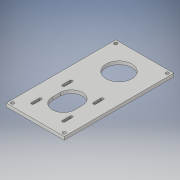
# Autodesk Inventor part: lid
Saved by Autodesk Inventor 2018 (Build 220112000, 112)
## iProperties
Created: 2018-07-04
Part Number: lid
Material: Generic
Document SubType Name: Modeling
Designer: Cole Tucker
Density: 1 g/cm^3
Appearance: Default
Author: Cole Tucker
Autodesk Inventor part; units mm, degrees
ref_plane "YZ Plane" through (0, 0, 0) normal (1, 0, 0) x (0, 1, 0)
ref_plane "XZ Plane" through (0, 0, 0) normal (0, 1, 0) x (-1, 0, 0)
ref_plane "XY Plane" through (0, 0, 0) normal (0, 0, 1) x (1, 0, 0)
sketch "Sketch1" plane through (0, 0, 0) normal (0, 1, 0) x (-1, 0, 0)
  line L0 (0, 0) -> (57.15, 0)
  line L1 (57.15, 0) -> (57.15, -107.95)
  line L2 (57.15, -107.95) -> (0, -107.95)
  line L3 (0, -107.95) -> (0, 0)
  line L4 (57.15, -53.975) -> (0, -53.975) construction
  circle A0 centre (28.575, -35.56) radius 11.049
  line L5 (28.575, -35.56) -> (43.815, -35.56) construction
  line L6 (43.815, -35.56) -> (43.815, -50.8) construction
  line L7 (43.815, -50.8) -> (28.575, -50.8) construction
  line L8 (28.575, -50.8) -> (28.575, -35.56) construction
  line L9 (28.575, -35.56) -> (13.335, -35.56) construction
  line L10 (13.335, -35.56) -> (13.335, -20.32) construction
  line L11 (13.335, -20.32) -> (28.575, -20.32) construction
  line L12 (28.575, -20.32) -> (28.575, -35.56) construction
  line L13 (43.815, -50.8) -> (13.335, -50.8) construction
  line L14 (13.335, -50.8) -> (13.335, -20.32) construction
  line L15 (13.335, -20.32) -> (43.815, -20.32) construction
  line L16 (43.815, -20.32) -> (43.815, -50.8) construction
  circle A1 centre (43.815, -50.8) radius 1.27
  circle A2 centre (43.815, -20.32) radius 1.27
  circle A3 centre (13.335, -50.8) radius 1.27
  circle A4 centre (13.335, -20.32) radius 1.27
  line L17 (28.575, -107.95) -> (28.575, -53.975) construction
  line L18 (28.575, -35.56) -> (28.575, -27.94) construction
  circle A5 centre (28.575, -27.94) radius 11.049
  line L19 (43.815, -50.8) -> (43.815, -43.18) construction
  line L20 (13.335, -50.8) -> (13.335, -43.18) construction
  line L21 (13.335, -20.32) -> (13.335, -12.7) construction
  line L22 (43.815, -20.32) -> (43.815, -12.7) construction
  circle A6 centre (43.815, -43.18) radius 1.27
  circle A7 centre (13.335, -43.18) radius 1.27
  circle A8 centre (13.335, -12.7) radius 1.27
  circle A9 centre (43.815, -12.7) radius 1.27
  line L23 (45.085, -43.18) -> (45.085, -50.8)
  line L24 (42.545, -43.18) -> (42.545, -50.8)
  line L25 (14.605, -43.18) -> (14.605, -50.8)
  line L26 (12.065, -43.18) -> (12.065, -50.8)
  line L27 (12.065, -12.7) -> (12.065, -20.32)
  line L28 (14.605, -20.32) -> (14.605, -12.7)
  line L29 (45.085, -12.7) -> (45.085, -20.32)
  line L30 (42.545, -20.32) -> (42.545, -12.7)
  line L31 (28.575, -107.95) -> (28.575, -82.55) construction
  circle A10 centre (28.575, -82.55) radius 12.7
  line L32 (57.15, 0) -> (57.15, -12.7)
  line L33 (57.15, 0) -> (44.45, 0)
  line L34 (44.45, 0) -> (57.15, -12.7) construction
  line L35 (57.15, 0) -> (50.8, -6.35) construction
  line L36 (0, 0) -> (12.7, 0) construction
  line L37 (0, 0) -> (0, -12.7) construction
  line L38 (0, -12.7) -> (12.7, 0) construction
  line L39 (0, 0) -> (6.35, -6.35) construction
  line L40 (57.15, -107.95) -> (57.15, -95.25) construction
  line L41 (57.15, -107.95) -> (44.45, -107.95) construction
  line L42 (44.45, -107.95) -> (57.15, -95.25) construction
  line L43 (57.15, -107.95) -> (50.8, -101.6) construction
  line L44 (0, -107.95) -> (12.7, -107.95) construction
  line L45 (0, -107.95) -> (0, -95.25) construction
  line L46 (0, -95.25) -> (12.7, -107.95) construction
  line L47 (6.35, -101.6) -> (0, -107.95) construction
  circle A11 centre (53.975, -104.775) radius 1.5875
  circle A12 centre (3.175, -104.775) radius 1.5875
  circle A13 centre (53.975, -3.175) radius 1.5875
  circle A14 centre (3.175, -3.175) radius 1.5875
  line L48 (17.526, -35.56) -> (17.526, -27.94)
  line L49 (39.624, -35.56) -> (39.624, -27.94)
  point P0 (38.7216, -23.5665)
  point P1 (18.4284, -23.5665)
  dimension "d0" = 57.15
  dimension "d1" = 107.95
  dimension "d2" = 22.098
  dimension "d3" = 15.24
  dimension "d4" = 15.24
  dimension "d5" = 15.24
  dimension "d6" = 15.24
  dimension "d7" = 2.54
  dimension "d8" = 2.54
  dimension "d9" = 2.54
  dimension "d10" = 2.54
  dimension "d11" = 7.62
  dimension "d12" = 22.098
  dimension "d13" = 7.62
  dimension "d14" = 7.62
  dimension "d15" = 7.62
  dimension "d16" = 7.62
  dimension "d17" = 2.54
  dimension "d18" = 2.54
  dimension "d19" = 2.54
  dimension "d20" = 2.54
  dimension "d21" = 25.4
  dimension "d22" = 25.4
  dimension "d25" = 12.7
  dimension "d26" = 12.7
  dimension "d27" = 12.7
  dimension "d28" = 12.7
  dimension "d29" = 12.7
  dimension "d30" = 12.7
  dimension "d31" = 12.7
  dimension "d32" = 12.7
  dimension "d33" = 3.175
  dimension "d34" = 3.175
  dimension "d35" = 3.175
  dimension "d36" = 3.175
  dimension "d39" = 35.56
  constraints: 100 end point, 22 point on circle, 19 point on line, 15 centre point, 13 midpoint, 13 parallel, 10 coincident, 6 perpendicular, 6 tangent, 4 horizontal, 3 vertical
  measures "d0" distance of L1.end L2.end
  measures "d1" distance of L0.end L1.end
  measures "d2" diameter of A0
  measures "d3" distance of L6.end L7.end
  measures "d4" distance of L5.end L6.end
  measures "d5" distance of L10.end L11.end
  measures "d6" distance of L9.end L10.end
  measures "d7" diameter of A1
  measures "d8" diameter of A2
  measures "d9" diameter of A3
  measures "d10" diameter of A4
  measures "d11" distance of L5.start L18.end
  measures "d12" diameter of A5
  measures "d13" distance of L19.start L19.end
  measures "d14" distance of L20.start L20.end
  measures "d15" distance of L21.start L21.end
  measures "d16" distance of L22.start L22.end
  measures "d17" diameter of A6
  measures "d18" diameter of A7
  measures "d19" diameter of A8
  measures "d20" diameter of A9
  measures "d21" distance of L17.start L31.end
  measures "d22" diameter of A10
  measures "d25" distance of L0.end L32.end
  measures "d26" distance of L0.end L33.end
  measures "d27" distance of L0.start L36.end
  measures "d28" distance of L0.start L37.end
  measures "d29" distance of L1.end L40.end
  measures "d30" distance of L1.end L41.end
  measures "d31" distance of L2.end L44.end
  measures "d32" distance of L2.end L45.end
  measures "d33" diameter of A11
  measures "d34" diameter of A12
  measures "d35" diameter of A13
  measures "d36" diameter of A14
  measures "d39" distance from line of L0 L5.start
extrude "Extrusion3" add sketch "Sketch1" along normal blind 3.175
equation "\"d3\" = d5"
equation "\"d4\" = d6"
equation "\"d7\" = d10"
equation "\"d8\" = d10"
equation "\"d9\" = d10"
equation "\"d12\" = d2"
equation "\"d13\" = d11"
equation "\"d14\" = d11"
equation "\"d15\" = d11"
equation "\"d16\" = d11"
equation "\"d17\" = d10"
equation "\"d18\" = d10"
equation "\"d19\" = d10"
equation "\"d20\" = d10"
body "Solid3"
